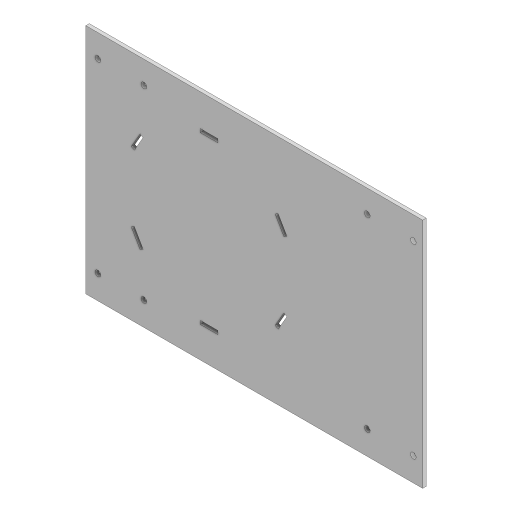
# Autodesk Inventor part: Base_final
Saved by Autodesk Inventor 2024 (Build 280153000, 153)
## iProperties
Created: 2024-04-13
Part Number: Base_final
Material: Generic
Document SubType Name: Modeling
Designer: op04o
Density: 1 g/cm^3
Appearance: Default
Author: op04o
Autodesk Inventor part; units mm, degrees
ref_plane "YZ Plane" through (0, 0, 0) normal (1, 0, 0) x (0, 1, 0)
ref_plane "XZ Plane" through (0, 0, 0) normal (0, 1, 0) x (-1, 0, 0)
ref_plane "XY Plane" through (0, 0, 0) normal (0, 0, 1) x (1, 0, 0)
sketch "Sketch1" plane through (0, 0, 0) normal (0, 0, 1) x (1, 0, 0)
  line L0 (173.1273, 69.5507) -> (165.6273, 56.5604)
  line L1 (165.6273, 56.5604) -> (163.0292, 58.0604)
  line L2 (163.0292, 58.0604) -> (170.5292, 71.0507)
  line L3 (170.5292, 71.0507) -> (173.1273, 69.5507)
  line L4 (113.6574, 26.5556) -> (98.6574, 26.5556)
  line L5 (98.6574, 26.5556) -> (98.6574, 29.5556)
  line L6 (98.6574, 29.5556) -> (113.6574, 29.5556)
  line L7 (113.6574, 29.5556) -> (113.6574, 26.5556)
  line L8 (46.6875, 142.5507) -> (49.2856, 141.0507)
  line L9 (49.2856, 141.0507) -> (41.7856, 128.0604)
  line L10 (41.7856, 128.0604) -> (39.1875, 129.5604)
  line L11 (39.1875, 129.5604) -> (46.6875, 142.5507)
  line L12 (46.6875, 56.5604) -> (39.1875, 69.5507)
  line L13 (39.1875, 69.5507) -> (41.7856, 71.0507)
  line L14 (41.7856, 71.0507) -> (49.2856, 58.0604)
  line L15 (49.2856, 58.0604) -> (46.6875, 56.5604)
  line L16 (98.6574, 172.5556) -> (113.6574, 172.5556)
  line L17 (113.6574, 172.5556) -> (113.6574, 169.5556)
  line L18 (113.6574, 169.5556) -> (98.6574, 169.5556)
  line L19 (98.6574, 169.5556) -> (98.6574, 172.5556)
  line L20 (165.6273, 142.5507) -> (173.1273, 129.5604)
  line L21 (173.1273, 129.5604) -> (170.5292, 128.0604)
  line L22 (170.5292, 128.0604) -> (163.0292, 141.0507)
  line L23 (163.0292, 141.0507) -> (165.6273, 142.5507)
  line L24 (290, 0) -> (290, 200)
  line L25 (290, 200) -> (0, 200)
  line L26 (0, 200) -> (0, 0)
  line L27 (0, 0) -> (290, 0)
  circle A0 centre (281.9574, 20.463) radius 2.5
  circle A1 centre (49.9574, 20.463) radius 2.5
  circle A2 centre (281.9574, 180.463) radius 2.5
  circle A3 centre (49.9574, 180.463) radius 2.5
  circle A4 centre (242.3574, 20.463) radius 2.5
  circle A5 centre (10.3574, 20.463) radius 2.5
  circle A6 centre (10.3574, 180.463) radius 2.5
  circle A7 centre (242.3574, 180.463) radius 2.5
  constraints: 56 end point, 8 centre point, 1 coincident
extrude "Extrusion1" add sketch "Sketch1" along normal blind 3
body "Solid1"
